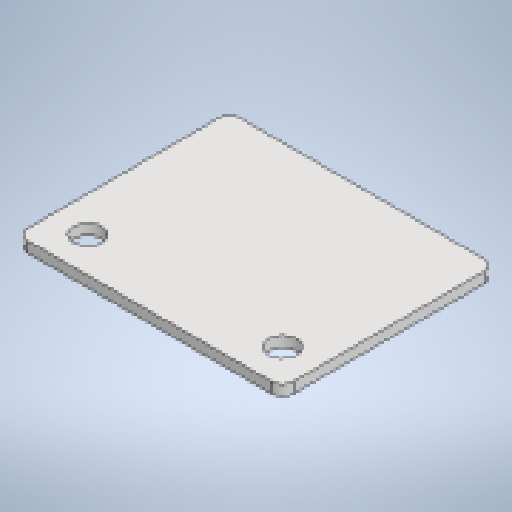
# Autodesk Inventor part: NDM-VOS pillar 2 plate 1
Saved by Autodesk Inventor 2025 (Build 290162010, 162A)
## iProperties
Created: 2025-11-09
Part Number: NDM-VOS pillar 2 plate 1
Material: Steel
Document SubType Name: Sheet Metal
Designer: admin
Stock Number: пластина опорная
Mass: 827.404 g
Surface Area: 389.153 cm^2
Volume: 105.402 cm^3
Density: 7.85 g/cm^3
Sheet Metal Rule: Default
Sheet Metal Width: 0.000 mm
Sheet Metal Length: 0.000 mm
Sheet Metal Area: 0.000 mm^2
Appearance: Default
Author: admin
Autodesk Inventor part; units mm, degrees
ref_plane "YZ Plane" through (0, 0, 0) normal (1, 0, 0) x (0, 1, 0)
ref_plane "XZ Plane" through (0, 0, 0) normal (0, 1, 0) x (-1, 0, 0)
ref_plane "XY Plane" through (0, 0, 0) normal (0, 0, 1) x (1, 0, 0)
sketch "Sketch1" plane through (0, 0, 0) normal (0, 0, 1) x (1, 0, 0)
  line L0 (-75, -60) -> (75, -60)
  line L1 (75, -60) -> (75, 60)
  line L2 (75, 60) -> (-75, 60)
  line L3 (-75, 60) -> (-75, -60)
  line L4 (-75, -60) -> (75, 60) construction
  line L5 (75, -60) -> (-75, 60) construction
  circle A0 centre (-55, 40) radius 8
  circle A1 centre (-55, -40) radius 8
  circle A2 centre (55, 40) radius 8
  circle A3 centre (55, -40) radius 8
  line L6 (0, 60) -> (0, -60) construction
  line L7 (-75, 0) -> (75, 0) construction
  point P0 (0, 0)
  dimension "d154" = 150
  dimension "d155" = 120
  dimension "d157" = 20
  dimension "d158" = 20
  dimension "d159" = 16
  measures "d154" distance of L1.end L2.end
  measures "d155" distance of L0.end L1.end
  measures "d157" distance from line of L2 A0.centre
  measures "d158" distance from line of L3 A0.centre
  measures "d159" diameter of A0
extrude "Plate5" add sketch "Sketch1" along normal blind 6 contours L3 L2 L1 L0 | A0 | A2
fillet "Corner Round1" radius 6 4 edges at (-75, -60, 3) (75, -60, 3) (75, 60, 3) (-75, 60, 3)
body "Solid3"
